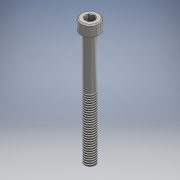
# Autodesk Inventor part: CB5-55
Saved by Autodesk Inventor 2016 (Build 200138000, 138)
## iProperties
Created: 2017-06-26
Part Number: CB5-55
Material: 鋼、炭素鋼
Document SubType Name: Modeling
Designer: yoguc
Density: 7.85 g/cm^3
Appearance: 半つや出し
Author: yoguc
Autodesk Inventor part; units mm, degrees
ref_plane "YZ Plane" through (0, 0, 0) normal (1, 0, 0) x (0, 1, 0)
ref_plane "XZ Plane" through (0, 0, 0) normal (0, 1, 0) x (-1, 0, 0)
ref_plane "XY Plane" through (0, 0, 0) normal (0, 0, 1) x (1, 0, 0)
sketch "スケッチ1" plane through (0, 0, 0) normal (1, 0, 0) x (0, 1, 0)
  line L0 (4.3, 5.1) -> (4.3, 0)
  line L1 (4.3, 0) -> (2.5, 0)
  line L2 (2.5, 0) -> (2.5, -55)
  line L3 (0, -55) -> (2.5, -55)
  line L4 (4.3, 5.1) -> (0, 5.1)
  line L5 (0, 5.1) -> (0, -55)
  point P0 (0, 0)
  dimension "d2" = 0
  dimension "d3" = 55
  dimension "d4" = 4.3
  dimension "d5" = 5.1
  dimension "d6" = 0
  dimension "d7" = 2.5
  constraints: 12 end point, 2 vertical, 1 horizontal, 1 perpendicular
  measures "d2" distance from line of point (0, 0) L1
  measures "d3" distance between parallel lines of L3 L1
  measures "d4" distance between parallel lines of L5 L0
  measures "d5" distance between parallel lines of L1 L4
  measures "d6" distance from line of point (0, 0) L5
  measures "d7" distance between parallel lines of L5 L2
revolve "回転1" add sketch "スケッチ1" angle 360 about axis through (0, 0, 5.1) along (0, 0, -1)
chamfer "面取り1" distance 0.5 angle 45 1 edges at (0, -4.3, 5.1)
sketch "スケッチ2" plane through (0, 0, 5.1) normal (0, 0, 1) x (1, 0, 0)
  circle A0 centre (0, 0) radius 2.29
  line L0 (0, 0) -> (-2.9175, 1.6844)
  line L1 (0, 0) -> (-1.7508, 0)
  point P0 (0, 0)
  point P1 (-1.9832, 1.145)
  point P2 (-1.9832, -1.145)
  point P3 (0, -2.29)
  point P4 (1.9832, -1.145)
  point P5 (1.9832, 1.145)
  point P6 (0, 2.29)
  dimension "d12" = 4.58
  dimension "d14" = 30
  dimension "d21" = 360
  constraints: 4 end point, 1 coincident, 1 horizontal, 1 point on line, 10 other
  measures "d14" angle of L1 L0
sketch "スケッチ3" plane through (0, 0, 5.1) normal (0, 0, 1) x (1, 0, 0)
  line L0 (-1.9832, 1.145) -> (0, 2.29)
  line L1 (0, 2.29) -> (1.9832, 1.145)
  line L2 (1.9832, 1.145) -> (1.9832, -1.145)
  line L3 (1.9832, -1.145) -> (0, -2.29)
  line L4 (0, -2.29) -> (-1.9832, -1.145)
  line L5 (-1.9832, -1.145) -> (-1.9832, 1.145)
  point P0 (0, 0)
  point P1 (-2.5, -1.3891)
  constraints: 12 end point, 3 parallel, 1 vertical
extrude "押し出し1" cut sketch "スケッチ3" against normal blind 4
thread "ねじ1" size "M6x1" class "6g" standard "ANSI Metric M Profile" length 30
sketch "スケッチ4" plane through (0, 0, 0) normal (0, 1, 0) x (-1, 0, 0)
  line L0 (-3.8, 5.1) -> (3.8, 5.1) projected
  line L1 (0, 5.1) -> (0, 1.1) projected
  line L2 (2.29, 5.1) -> (1.9832, 4.7932)
  line L3 (1.9832, 5.1) -> (1.9832, 1.1) projected
  line L4 (1.9832, 5.1) -> (2.29, 5.1)
  point P0 (0, 0)
  dimension "d27" = 2.29
  dimension "d28" = 45
  constraints: 4 end point, 2 point on line, 1 perpendicular
  measures "d27" distance from line of L1 L2.start
  measures "d28" angle of L3 L2
revolve "回転2" cut sketch "スケッチ4" angle 360 about axis through (0, 0, 5.1) along (0, 0, -1)
